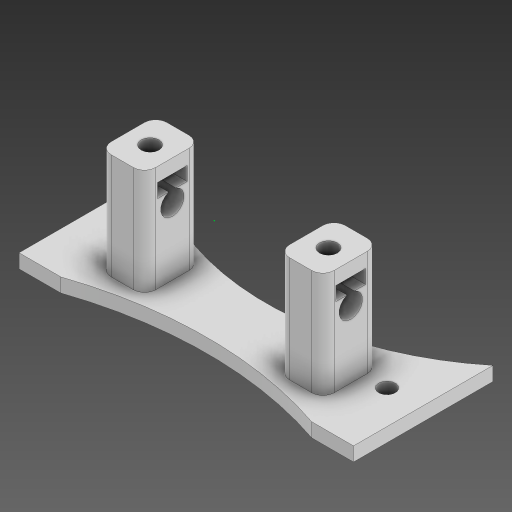
# Autodesk Inventor part: kreplenie_dribler
Saved by Autodesk Inventor 2023 (Build 270158000, 158)
## iProperties
Created: 2025-05-24
Part Number: kreplenie_dribler
Material: Типовые
Document SubType Name: Modeling
Designer: daa
Density: 1 g/cm^3
Appearance: По умолчанию
Author: daa
Autodesk Inventor part; units mm, degrees
ref_plane "YZ Plane" through (0, 0, 0) normal (1, 0, 0) x (0, 1, 0)
ref_plane "XZ Plane" through (0, 0, 0) normal (0, 1, 0) x (-1, 0, 0)
ref_plane "XY Plane" through (0, 0, 0) normal (0, 0, 1) x (1, 0, 0)
sketch "Эскиз1" plane through (0, 0, 0) normal (0, 1, 0) x (-1, 0, 0)
  arc A0 (-52.5, 25) -> (-7.5, 25) centre (-30, 91.2854) ccw
  arc A1 (0, 0) -> (-60, 0) centre (-30, -36.8273) ccw
  circle A2 centre (-54, 13) radius 1.5
  circle A3 centre (-6.289, 13) radius 1.5
  line L0 (-7.5, 25) -> (0, 25)
  line L1 (-52.5, 25) -> (-60, 25)
  line L2 (0, 25) -> (0, 0)
  line L3 (-60, 25) -> (-60, 0)
  dimension "d4" = 45
  dimension "d8" = 70
  dimension "d9" = 47.5
  dimension "d10" = 3
  dimension "d11" = 3
  dimension "d12" = 47.711
  dimension "d15" = 13
  dimension "d16" = 13
  dimension "d87" = 6.289
  constraints: 8 end point, 4 centre point, 4 point on circle, 1 parallel, 1 point on line, 1 vertical
  measures "d4" distance of L0.start L1.start
  measures "d8" radius of A0
  measures "d9" radius of A1
  measures "d10" diameter of A2
  measures "d11" diameter of A3
  measures "d12" distance of A3.centre A2.centre
  measures "d15" vertical distance of L2.end A3.centre
  measures "d16" vertical distance of A2.centre L3.end
  measures "d87" distance from line of L2 A3.centre
extrude "Выдавливание1" add sketch "Эскиз1" along normal blind 2.5
sketch "Эскиз2" plane through (0, 2.5, 0) normal (0, 1, 0) x (1, 0, 0)
  line L0 (42, -20.5) -> (50, -20.5)
  line L1 (50, -20.5) -> (50, -10.5)
  line L2 (50, -10.5) -> (42, -10.5)
  line L3 (42, -10.5) -> (42, -20.5)
  circle A0 centre (54, -13) radius 1.5 projected
  line L4 (10, -20.5) -> (18, -20.5)
  line L5 (18, -20.5) -> (18, -10.5)
  line L6 (18, -10.5) -> (10, -10.5)
  line L7 (10, -10.5) -> (10, -20.5)
  circle A1 centre (6.289, -13) radius 1.5 projected
  circle A2 centre (6.289, -13) radius 2.75
  line L8 (0, 0) -> (0, -25) projected
  line L9 (60, -25) -> (60, 0) projected
  point P0 (7.5, -25)
  point P1 (52.5, -40)
  point P2 (14, -20.5)
  dimension "d28" = 8
  dimension "d29" = 10
  dimension "d32" = 8
  dimension "d33" = 10
  dimension "d44" = 5.5
  dimension "d45" = 10
  dimension "d46" = 10
  dimension "d47" = 4.5
  dimension "d48" = 4.5
  constraints: 16 end point, 4 parallel, 2 horizontal, 2 perpendicular, 1 centre point, 1 coincident, 1 midpoint
  measures "d28" distance of L2.end L1.end
  measures "d29" distance of L1.end L0.end
  measures "d32" distance of L6.end L5.end
  measures "d33" distance of L5.end L4.end
  measures "d44" diameter of A2
  measures "d45" distance between parallel lines of L7 L8
  measures "d46" distance between parallel lines of L9 L1
  measures "d47" vertical distance of L0.end L9.start
  measures "d48" vertical distance of L4.start L8.end
extrude "Выдавливание2" add sketch "Эскиз2" along normal blind 19 contours L3 L2 L1 L0 | L7 L6 L5 L4
fillet "Сопряжение1" radius 2 8 edges at (50, 12, 20.5) (50, 12, 10.5) (42, 12, 20.5) (42, 12, 10.5) (10, 12, 10.5) (18, 12, 10.5) (18, 12, 20.5) (10, 12, 20.5)
sketch "Эскиз4" plane through (50, 2.5, 18.5) normal (1, 0, 0) x (0, 0, -1)
  circle A0 centre (3, 12) radius 2.1
  line L0 (6, 19) -> (6, 0) projected
  line L1 (-6.5, 0) -> (18.5, 0) projected
  point P0 (18.5, -2.5)
  dimension "d39" = 4.2
  dimension "d40" = 3
  dimension "d41" = 12
  constraints: 1 centre point
  measures "d39" diameter of A0
  measures "d40" distance from line of L0 A0.centre
  measures "d41" distance from line of L1 A0.centre
extrude "Выдавливание4" cut sketch "Эскиз4" against normal blind 49
sketch "Эскиз9" plane through (0, 21.5, 0) normal (0, 1, 0) x (1, 0, 0)
  circle A0 centre (46, -15.5) radius 1.6
  circle A1 centre (14, -15.5) radius 1.6
  line L0 (42, -12.5) -> (42, -18.5) projected
  line L1 (44, -20.5) -> (48, -20.5) projected
  line L2 (18, -18.5) -> (18, -12.5) projected
  line L3 (12, -20.5) -> (16, -20.5) projected
  point P0 (0, 0)
  point P1 (42, -15.5)
  point P2 (46, -20.5)
  dimension "d73" = 3.2
  dimension "d74" = 3.2
  dimension "d75" = 4
  dimension "d76" = 5
  dimension "d77" = 4
  dimension "d78" = 5
  constraints: 2 centre point, 2 midpoint
  measures "d73" diameter of A0
  measures "d74" diameter of A1
  measures "d75" distance of point (42, -15.5) A0.centre
  measures "d76" distance of point (46, -20.5) A0.centre
  measures "d77" distance from line of A1.centre L2
  measures "d78" distance from line of L3 A1.centre
extrude "Выдавливание9" cut sketch "Эскиз9" against normal blind 6
sketch "Эскиз10" plane through (50, 2.5, 18.5) normal (1, 0, 0) x (0, 0, -1)
  line L0 (0.35, 16.5) -> (5.65, 16.5)
  line L1 (5.65, 16.5) -> (5.65, 14)
  line L2 (5.65, 14) -> (0.35, 14)
  line L3 (0.35, 14) -> (0.35, 16.5)
  line L4 (0, 19) -> (6, 19) projected
  line L5 (0, 0) -> (0, 19) projected
  point P0 (18.5, -2.5)
  dimension "d81" = 5.3
  dimension "d82" = 2.5
  dimension "d83" = 2.5
  dimension "d84" = 0.35
  constraints: 8 end point, 2 parallel, 1 horizontal, 1 perpendicular
  measures "d81" distance of L1.end L2.end
  measures "d82" distance of L0.end L1.end
  measures "d83" distance between parallel lines of L4 L0
  measures "d84" distance between parallel lines of L3 L5
extrude "Выдавливание10" cut sketch "Эскиз10" against normal blind 54.25
sketch "Эскиз11" plane through (10, 2.5, 12.5) normal (-1, 0, 0) x (0, 0, 1)
  point P0 (-12.5, -2.5)
